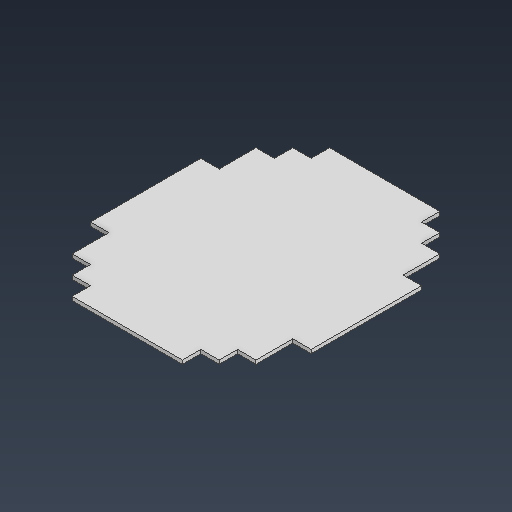
# Autodesk Inventor part: Shell
Saved by Autodesk Inventor 2025.3 (Build 293356000, 356)
## iProperties
Created: 2026-01-26
Part Number: Shell
Material: Generic
Document SubType Name: Modeling
Designer: tolga
Density: 1 g/cm^3
Appearance: Default
Author: tolga
Autodesk Inventor part; units mm, degrees
ref_plane "YZ Plane" through (0, 0, 0) normal (1, 0, 0) x (0, 1, 0)
ref_plane "XZ Plane" through (0, 0, 0) normal (0, 1, 0) x (-1, 0, 0)
ref_plane "XY Plane" through (0, 0, 0) normal (0, 0, 1) x (1, 0, 0)
sketch "Sketch1" plane through (0, 0, 0) normal (0, 1, 0) x (-1, 0, 0)
  line L0 (0, 0) -> (30, 0)
  line L1 (30, 0) -> (30, -10)
  line L2 (30, -10) -> (40, -10)
  line L3 (40, -10) -> (40, -20)
  line L4 (40, -20) -> (50, -20)
  line L5 (50, -20) -> (50, -40)
  line L6 (50, -40) -> (60, -40)
  line L7 (60, -40) -> (60, -70)
  line L8 (0, 0) -> (0, -70) construction
  line L9 (60, -70) -> (0, -70) construction
  line L10 (0, -140) -> (30, -140)
  line L11 (30, -140) -> (30, -130)
  line L12 (30, -130) -> (40, -130)
  line L13 (40, -130) -> (40, -120)
  line L14 (40, -120) -> (50, -120)
  line L15 (50, -120) -> (50, -100)
  line L16 (50, -100) -> (60, -100)
  line L17 (60, -100) -> (60, -70)
  line L18 (0, 0) -> (-30, 0)
  line L19 (-30, 0) -> (-30, -10)
  line L20 (-30, -10) -> (-40, -10)
  line L21 (-40, -10) -> (-40, -20)
  line L22 (-40, -20) -> (-50, -20)
  line L23 (-50, -20) -> (-50, -40)
  line L24 (-50, -40) -> (-60, -40)
  line L25 (-60, -40) -> (-60, -70)
  line L26 (0, -140) -> (-30, -140)
  line L27 (-30, -140) -> (-30, -130)
  line L28 (-30, -130) -> (-40, -130)
  line L29 (-40, -130) -> (-40, -120)
  line L30 (-40, -120) -> (-50, -120)
  line L31 (-50, -120) -> (-50, -100)
  line L32 (-50, -100) -> (-60, -100)
  line L33 (-60, -100) -> (-60, -70)
  dimension "d0" = 10
  dimension "d1" = 30
  dimension "d2" = 10
  dimension "d3" = 10
  dimension "d4" = 20
  dimension "d5" = 30
  dimension "d6" = 10
  dimension "d7" = 10
  constraints: 68 end point, 23 symmetric about line, 6 perpendicular, 3 horizontal, 1 vertical
  measures "d0" distance of L0.end L1.end
  measures "d1" distance of L0.start L0.end
  measures "d2" distance of L2.end L3.end
  measures "d3" distance of L1.end L2.end
  measures "d4" distance of L4.end L5.end
  measures "d5" distance of L6.end L7.end
  measures "d6" distance of L3.end L4.end
  measures "d7" distance of L5.end L6.end
extrude "Extrusion1" add sketch "Sketch1" along normal blind 2
equation "\"d1\" = 3 * d0"
equation "\"d2\" = d0"
equation "\"d3\" = d0"
equation "\"d4\" = 2 * d0"
equation "\"d5\" = 3 * d0"
equation "\"d6\" = d0"
equation "\"d7\" = d0"
body "Solid1"
